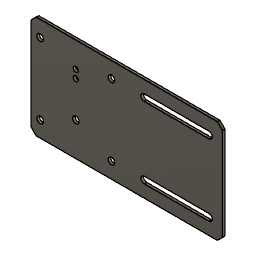
_Tensioner and Idler Mount.bc5086e5-d5f1-4108-8d36-0b39635d839e (Autodesk Fusion 360 design; units mm, degrees)
Autodesk Fusion 360 part; units mm, degrees
sketch "Sketch1" plane through (0, 0, 0) normal (0, 0, 1) x (1, 0, 0)
  circle A0 centre (79, 15.5) radius 3.2
  arc A1 (111.2, 18.7) -> (111.2, 12.3) centre (111.2, 15.5) ccw
  line L0 (111.2, 15.5) -> (174.8, 15.5) construction
  arc A2 (174.8, 12.3) -> (174.8, 18.7) centre (174.8, 15.5) ccw
  line L1 (111.2, 85.5) -> (174.8, 85.5) construction
  arc A3 (111.2, 88.7) -> (111.2, 82.3) centre (111.2, 85.5) ccw
  circle A4 centre (44, 50.5) radius 36.5 construction
  line L2 (188, 0) -> (188, 101)
  line L3 (111.2, 82.3) -> (174.8, 82.3)
  line L4 (0, 50.5) -> (188, 50.5) construction
  line L5 (188, 101) -> (0, 101)
  line L6 (9, 15.5) -> (9, 85.5) construction
  arc A5 (174.8, 82.3) -> (174.8, 88.7) centre (174.8, 85.5) ccw
  line L7 (111.2, 12.3) -> (174.8, 12.3)
  line L8 (79, 15.5) -> (9, 15.5) construction
  circle A6 centre (9, 85.5) radius 3.2
  line L9 (79, 85.5) -> (79, 15.5) construction
  line L10 (9, 85.5) -> (79, 85.5) construction
  circle A7 centre (79, 85.5) radius 3.2
  circle A8 centre (9, 15.5) radius 3.2
  line L11 (0, 0) -> (188, 0)
  line L12 (174.8, 18.7) -> (111.2, 18.7)
  line L13 (0, 101) -> (0, 0)
  line L14 (174.8, 88.7) -> (111.2, 88.7)
  line L15 (44, 50.5) -> (44, 68) construction
  line L16 (44, 68) -> (44, 76) construction
  line L17 (44, 50.5) -> (44, 33) construction
  circle A9 centre (44, 76) radius 2.5
  circle A10 centre (44, 68) radius 2.5
  circle A11 centre (44, 33) radius 3.2
  point P0 (44, 85.5)
  point P1 (9, 50.5)
  point P2 (178, 85.5)
  point P3 (108, 85.5)
  dimension "d1" = 188
  dimension "d2" = 101
  dimension "d3" = 73
  dimension "d4" = 70
  dimension "d5" = 6.4
  dimension "d6" = 9
  dimension "d7" = 10
  dimension "d8" = 70
  dimension "d9" = 17.5
  dimension "d10" = 8
  dimension "d11" = 17.5
  dimension "d12" = 5
  dimension "d13" = 5
  dimension "d14" = 6.4
  constraint horizontal L11
  constraint vertical L2
  constraint horizontal L5
  constraint vertical L13
  constraint coincident L11.start L13.end
  constraint midpoint L4.start L13
  constraint midpoint L4.end L2
  constraint coincident A4.centre L4
  constraint horizontal L10
  constraint vertical L9
  constraint horizontal L8
  constraint vertical L6
  constraint equal L6 L10
  constraint midpoint P0 L10
  constraint vertical P0 A4.centre
  constraint midpoint P1 L6
  constraint horizontal P1 A4.centre
  constraint coincident L6.end A6.centre
  constraint coincident L9.start L10.end
  constraint coincident A0.centre L8.start
  constraint coincident L6.start L8.end
  constraint equal A0 A8
  constraint equal A0 A7
  constraint equal A6 A7
  constraint tangent A2 L7
  constraint tangent A2 L12
  constraint parallel L7 L12
  constraint tangent A1 L12
  constraint tangent A1 L7
  constraint horizontal L0
  constraint tangent L3 A5
  constraint tangent A5 L14
  constraint parallel L3 L14
  constraint tangent A3 L14
  constraint tangent A3 L3
  constraint parallel L1 L12
  constraint equal A5 A7
  constraint equal A0 A2
  constraint coincident A0.centre L0
  constraint coincident L9.start L1
  constraint equal L0 L1
  constraint midpoint P2 A5
  constraint vertical L1.end L0.end
  constraint midpoint P3 A3
  constraint coincident A4.centre L15.start
  constraint perpendicular L4 L15
  constraint parallel L15 L16
  constraint perpendicular L4 L17
  constraint coincident L16.end A9.centre
  constraint coincident L15.end L16.start
  constraint coincident L17.end A11.centre
  measures "d1" distance of L2.start L11.start
  measures "d2" distance of L5.end L11.start
  measures "d3" diameter of A4
  measures "d4" distance of L6.end L6.start
  measures "d5" diameter of A6
  measures "d6" distance of L6.start L13
  measures "d7" distance of P2 L2
  measures "d8" distance of P2 P3
  measures "d9" distance of A4.centre L15.end
  measures "d10" distance of L15.end L16.end
  measures "d11" distance of A4.centre L17.end
  measures "d12" diameter of A9
  measures "d13" diameter of A10
  measures "d14" diameter of A11
extrude "BaseFlange1" add sketch "Sketch1" along normal blind 2.5
chamfer "Chamfer1" distance 5 angle 45 4 edges at (0, 101, 1.25) (188, 101, 1.25) (188, 0, 1.25) (0, 0, 1.25)
